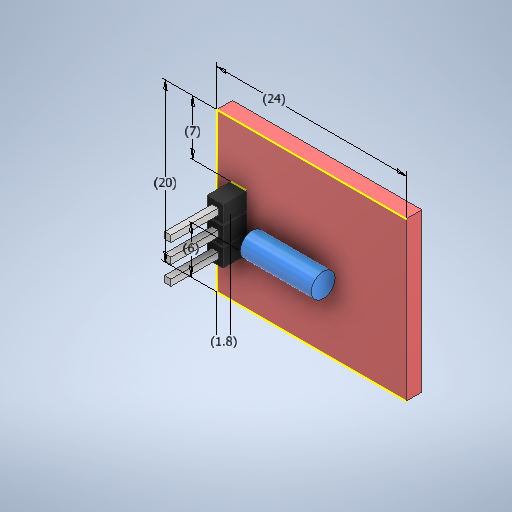
# Autodesk Inventor part: SecondCircuit
Saved by Autodesk Inventor 2025.1 (Build 291241020, 241B)
## iProperties
Created: 2024-08-30
Part Number: SecondCircuit
Material: Generic
Document SubType Name: Modeling
Designer: andre
Density: 1 g/cm^3
Appearance: Default
Author: andre
Autodesk Inventor part; units mm, degrees
ref_plane "YZ Plane" through (0, 0, 0) normal (1, 0, 0) x (0, 1, 0)
ref_plane "XZ Plane" through (0, 0, 0) normal (0, 1, 0) x (-1, 0, 0)
ref_plane "XY Plane" through (0, 0, 0) normal (0, 0, 1) x (1, 0, 0)
sketch "Sketch1" plane through (0, 0, 0) normal (0, 0, 1) x (1, 0, 0)
  line L0 (0, 0) -> (24, 0)
  line L1 (24, 0) -> (24, 20)
  line L2 (24, 20) -> (0, 20)
  line L3 (0, 20) -> (0, 0)
  dimension "d0" = 24
  dimension "d1" = 20
  constraints: 8 end point, 2 parallel, 1 horizontal, 1 perpendicular
  measures "d0" distance of L1.end L2.end
  measures "d1" distance of L0.end L1.end
extrude "Extrusion1" add sketch "Sketch1" along normal blind 2
ref_plane "Work Plane1" through (15, 0, 0) normal (1, 0, 0) x (0, 0, -1)
sketch "Sketch2" plane through (15, 0, 0) normal (1, 0, 0) x (0, 0, -1)
  circle A0 centre (-3.5, 9) radius 1.5
  line L0 (-2, 0) -> (-2, 20) projected
  line L1 (0, 0) -> (-2, 0) projected
  dimension "d5" = 3
  dimension "d6" = 9
  constraints: 1 centre point, 1 tangent
  measures "d5" diameter of A0
  measures "d6" distance from line of L1 A0.centre
extrude "Extrusion2" add sketch "Sketch2" against normal blind 9
sketch "Sketch3" plane through (0, 0, 2) normal (0, 0, 1) x (1, 0, 0)
  point P0 (0, 0)
sketch "Sketch4" plane through (0, 0, 2) normal (0, 0, 1) x (1, 0, 0)
  line L0 (1.8, 13) -> (3.8, 13)
  line L1 (3.8, 13) -> (3.8, 10.8)
  line L2 (3.8, 10.8) -> (1.8, 10.8)
  line L3 (1.8, 10.8) -> (1.8, 13)
  line L4 (1.8, 10.6) -> (3.8, 10.6)
  line L5 (3.8, 10.6) -> (3.8, 8.4)
  line L6 (3.8, 8.4) -> (1.8, 8.4)
  line L7 (1.8, 8.4) -> (1.8, 10.6)
  line L8 (1.8, 8.2) -> (3.8, 8.2)
  line L9 (3.8, 8.2) -> (3.8, 6)
  line L10 (3.8, 6) -> (1.8, 6)
  line L11 (1.8, 6) -> (1.8, 8.2)
  line L12 (24, 0) -> (24, 20) projected
  line L13 (0, 0) -> (24, 0) projected
  line L14 (0, 20) -> (0, 0) projected
  line L15 (24, 20) -> (0, 20) projected
  point P0 (2.8, 10.8)
  dimension "d11" = 2
  dimension "d12" = 2.2
  dimension "d13" = 2
  dimension "d14" = 2.2
  dimension "d15" = 2
  dimension "d16" = 2.2
  dimension "d26" = 0.2
  dimension "d27" = 0.2
  dimension "d28" = 1.8
  dimension "d60" = 7
  constraints: 24 end point, 6 parallel, 3 horizontal, 3 perpendicular, 2 vertical alignment, 1 midpoint
  measures "d11" distance of L1.end L2.end
  measures "d12" distance of L0.end L1.end
  measures "d13" distance of L5.end L6.end
  measures "d14" distance of L4.end L5.end
  measures "d15" distance of L9.end L10.end
  measures "d16" distance of L8.end L9.end
  measures "d26" distance between parallel lines of L6 L8
  measures "d27" distance from line of point (2.8, 10.8) L4
  measures "d28" distance between parallel lines of L14 L3
  measures "d60" distance between parallel lines of L15 L0
extrude "Extrusion3" add sketch "Sketch4" along normal blind 3 contours L0 L1 L2 L3 | L4 L5 L6 L7 | L8 L9 L10 L11
sketch "Sketch6" plane through (0, 0, 5) normal (0, 0, 1) x (1, 0, 0)
  line L0 (1.8, 10.8) -> (3.8, 10.8) projected
  line L1 (3.8, 10.8) -> (3.8, 13) projected
  line L2 (3.8, 13) -> (1.8, 13) projected
  line L3 (1.8, 13) -> (1.8, 10.8) projected
  line L4 (1.8, 8.4) -> (3.8, 8.4) projected
  line L5 (3.8, 8.4) -> (3.8, 10.6) projected
  line L6 (3.8, 10.6) -> (1.8, 10.6) projected
  line L7 (1.8, 10.6) -> (1.8, 8.4) projected
  line L8 (1.8, 6) -> (3.8, 6) projected
  line L9 (3.8, 6) -> (3.8, 8.2) projected
  line L10 (3.8, 8.2) -> (1.8, 8.2) projected
  line L11 (1.8, 8.2) -> (1.8, 6) projected
  line L12 (2.4, 12.3) -> (3.2, 12.3)
  line L13 (3.2, 12.3) -> (3.2, 11.5)
  line L14 (3.2, 11.5) -> (2.4, 11.5)
  line L15 (2.4, 11.5) -> (2.4, 12.3)
  line L16 (2.4, 9.9) -> (3.2, 9.9)
  line L17 (3.2, 9.9) -> (3.2, 9.1)
  line L18 (3.2, 9.1) -> (2.4, 9.1)
  line L19 (2.4, 9.1) -> (2.4, 9.9)
  line L20 (2.4, 7.5) -> (3.2, 7.5)
  line L21 (3.2, 7.5) -> (3.2, 6.7)
  line L22 (3.2, 6.7) -> (2.4, 6.7)
  line L23 (2.4, 6.7) -> (2.4, 7.5)
  line L24 (3.8, 13) -> (1.8, 13) projected
  point P0 (0, 0)
  point P1 (2.8, 9.9)
  point P2 (2.8, 13)
  point P3 (2.8, 7.5)
  point P4 (2.8, 13)
  point P5 (2.8, 12.3)
  point P6 (2.8, 8.4)
  point P7 (2.4, 11.9)
  point P8 (1.8, 11.9)
  point P9 (2.4, 9.5)
  point P10 (1.8, 9.5)
  point P11 (2.4, 7.1)
  point P12 (1.8, 7.1)
  dimension "d45" = 0.8
  dimension "d46" = 0.8
  dimension "d47" = 0.8
  dimension "d48" = 0.8
  dimension "d49" = 0.8
  dimension "d50" = 0.8
  constraints: 24 end point, 12 midpoint, 6 parallel, 3 horizontal, 3 horizontal alignment, 3 perpendicular, 3 vertical alignment
  measures "d45" distance of L13.end L14.end
  measures "d46" distance of L12.end L13.end
  measures "d47" distance of L18.start L18.end
  measures "d48" distance of L16.end L18.start
  measures "d49" distance of L22.start L22.end
  measures "d50" distance of L20.end L22.start
extrude "Extrusion5" add sketch "Sketch6" along normal blind 6 contours L12 L13 L14 L15 | L16 L17 L18 L19 | L20 L21 L22 L23
sketch "Sketch9" plane through (0, 0, 2) normal (0, 0, 1) x (1, 0, 0)
  line L0 (24, 20) -> (0, 20) projected
  line L1 (3.8, 13) -> (1.8, 13) projected
  line L2 (0, 0) -> (24, 0) projected
  line L3 (1.8, 6) -> (3.8, 6) projected
  line L4 (0, 20) -> (0, 0) projected
  line L5 (1.8, 10.6) -> (1.8, 8.4) projected
  point P0 (2.8, 6)
  point P1 (1.8, 9.5)
  dimension "d61" = 7
  dimension "d62" = 6
  dimension "d63" = 1.8
  dimension "d64" = 24
  dimension "d65" = 20
  constraints: 2 midpoint
  measures "d61" distance between parallel lines of L0 L1
  measures "d62" distance from line of L2 point (2.8, 6)
  measures "d63" distance from line of L4 point (1.8, 9.5)
  measures "d64" distance of L0.start L0.end
  measures "d65" distance of L0.end L2.start
body "Solid1"
